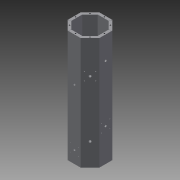
# Autodesk Inventor part: CentralRod_v1.2
Saved by Autodesk Inventor 2015 (Build 190159000, 159)
## iProperties
Created: 2015-09-24
Part Number: CentralRod_v1.2
Material: Generic
Document SubType Name: Modeling
Designer: Stefania
Density: 1 g/cm^3
Appearance: Default
Author: Stefania
Autodesk Inventor part; units mm, degrees
note: some values were not read from the file. Chosen so that the rebuilt part matches the saved one: kept side of "Split6".
ref_plane "XZ Plane" through (0, 0, 0) normal (0, 1, 0) x (-1, 0, 0)
ref_plane "XY Plane" through (0, 0, 0) normal (0, 0, 1) x (1, 0, 0)
sketch "Sketch1" plane through (0, 0, 0) normal (0, 0, 1) x (1, 0, 0)
  line L0 (-15.367, 37.0992) -> (15.367, 37.0992)
  line L1 (15.367, 37.0992) -> (37.0992, 15.367)
  line L2 (37.0992, 15.367) -> (37.0992, -15.367)
  line L3 (37.0992, -15.367) -> (15.367, -37.0992)
  line L4 (15.367, -37.0992) -> (-15.367, -37.0992)
  line L5 (-15.367, -37.0992) -> (-37.0992, -15.367)
  line L6 (-37.0992, -15.367) -> (-37.0992, 15.367)
  line L7 (-37.0992, 15.367) -> (-15.367, 37.0992)
  line L8 (-18.5233, 44.7192) -> (18.5233, 44.7192)
  line L9 (18.5233, 44.7192) -> (44.7192, 18.5233)
  line L10 (44.7192, 18.5233) -> (44.7192, -18.5233)
  line L11 (44.7192, -18.5233) -> (18.5233, -44.7192)
  line L12 (18.5233, -44.7192) -> (-18.5233, -44.7192)
  line L13 (-18.5233, -44.7192) -> (-44.7192, -18.5233)
  line L14 (-44.7192, -18.5233) -> (-44.7192, 18.5233)
  line L15 (-44.7192, 18.5233) -> (-18.5233, 44.7192)
  point P0 (0, 0)
  point P1 (0, 0)
  point P2 (-37.0992, 0)
  point P3 (0, 37.0992)
  dimension "d0" = 30.734
  dimension "d1" = 7.62
  constraints: 32 end point, 2 midpoint, 1 coincident, 1 horizontal alignment, 1 vertical alignment, 24 other
  measures "d0" distance of L0.start L0.end
  measures "d1" distance between parallel lines of L7 L15
extrude "Extrusion1" add sketch "Sketch1" along normal mid plane 304.8
sketch "Sketch2" plane through (18.5233, 44.7192, 152.4) normal (0.7071068, 0.7071068, 0) x (0, 0, -1)
  circle A0 centre (28.956, -18.5233) radius 3.175
  line L0 (0, -37.0466) -> (0, 0) projected
  circle A1 centre (188.976, -18.5233) radius 3.175
  line L1 (304.8, 0) -> (304.8, -37.0466) projected
  point P0 (152.4, -18.5233)
  dimension "d4" = 6.35
  dimension "d5" = 28.956
  dimension "d6" = 6.35
  dimension "d7" = 115.824
  constraints: 2 centre point
  measures "d4" diameter of A0
  measures "d5" distance from line of L0 A0.centre
  measures "d6" diameter of A1
  measures "d7" distance from line of A1.centre L1
extrude "Extrusion2" cut sketch "Sketch2" against normal through all
sketch "Sketch3" plane through (44.7192, -18.5233, 152.4) normal (1, 0, 0) x (0, 0, -1)
  circle A0 centre (57.912, 18.5233) radius 3.175
  line L0 (0, 0) -> (0, 37.0466) projected
  circle A1 centre (217.932, 18.5233) radius 3.175
  point P0 (152.4, 18.5233)
  dimension "d10" = 6.35
  dimension "d11" = 57.912
  dimension "d12" = 6.35
  dimension "d13" = 160.02
  constraints: 2 centre point
  measures "d10" diameter of A0
  measures "d11" distance from line of L0 A0.centre
  measures "d12" diameter of A1
  measures "d13" distance of A1.centre A0.centre
extrude "Extrusion3" cut sketch "Sketch3" against normal through all
sketch "Sketch4" plane through (44.7192, -18.5233, -152.4) normal (0.7071068, -0.7071068, 0) x (0.7071068, 0.7071068, 0)
  circle A0 centre (-18.5233, 217.932) radius 3.175
  line L0 (-37.0466, 304.8) -> (0, 304.8) projected
  circle A1 centre (-18.5233, 57.912) radius 3.175
  point P0 (-18.5233, 152.4)
  dimension "d16" = 6.35
  dimension "d17" = 86.868
  dimension "d18" = 6.35
  dimension "d19" = 160.02
  constraints: 2 centre point
  measures "d16" diameter of A0
  measures "d17" distance from line of L0 A0.centre
  measures "d18" diameter of A1
  measures "d19" distance of A1.centre A0.centre
extrude "Extrusion4" cut sketch "Sketch4" against normal through all
sketch "Sketch5" plane through (-18.5233, -44.7192, 152.4) normal (0, -1, 0) x (1, 0, 0)
  circle A0 centre (18.5233, -115.824) radius 3.175
  circle A1 centre (18.5233, -275.844) radius 3.175
  line L0 (0, 0) -> (37.0466, 0) projected
  point P0 (18.5233, -152.4)
  dimension "d22" = 6.35
  dimension "d23" = 6.35
  dimension "d24" = 115.824
  dimension "d25" = 160.02
  constraints: 2 centre point
  measures "d22" diameter of A0
  measures "d23" diameter of A1
  measures "d24" distance from line of L0 A0.centre
  measures "d25" distance of A1.centre A0.centre
extrude "Extrusion5" cut sketch "Sketch5" against normal through all
sketch "Sketch6" plane through (18.5233, 44.7192, 152.4) normal (0.7071068, 0.7071068, 0) x (0, 0, -1)
  circle A0 centre (17.399, -6.9663) radius 1.016
  circle A1 centre (28.956, -18.5233) radius 3.175 projected
  line L0 (0, 0) -> (304.8, 0) projected
  line L1 (0, -37.0466) -> (0, 0) projected
  circle A2 centre (17.399, -30.0803) radius 1.016
  circle A3 centre (40.513, -6.9663) radius 1.016
  circle A4 centre (40.513, -30.0803) radius 1.016
  point P0 (152.4, -18.5233)
  dimension "d28" = 2.032
  dimension "d29" = 11.557
  dimension "d30" = 11.557
  dimension "d33" = 23.114
  dimension "d40" = 23.114
  constraints: 4 centre point, 1 horizontal, 1 vertical, 6 other
  measures "d28" diameter of A0
  measures "d29" horizontal distance of A1.centre A0.centre
  measures "d30" horizontal distance of A0.centre A1.centre
  measures "d33" distance of A0.centre A2.centre
  measures "d40" distance of A0.centre A3.centre
extrude "Extrusion6" cut sketch "Sketch6" against normal up to surface (7.62 mm away) contours A0 | A2 | A3 | A4
sketch "Sketch7" plane through (-18.5233, -44.7192, -152.4) normal (-0.7071068, -0.7071068, 0) x (0, 0, 1)
  circle A0 centre (127.381, 30.0803) radius 1.016
  circle A1 centre (115.824, 18.5233) radius 3.175 projected
  line L0 (304.8, 37.0466) -> (0, 37.0466) projected
  line L1 (0, 0) -> (0, 37.0466) projected
  circle A2 centre (104.267, 30.0803) radius 1.016
  circle A3 centre (127.381, 6.9663) radius 1.016
  circle A4 centre (104.267, 6.9663) radius 1.016
  point P0 (152.4, 18.5233)
  dimension "d47" = 2.032
  dimension "d48" = 11.557
  dimension "d49" = 11.557
  dimension "d52" = 23.114
  dimension "d59" = 23.114
  constraints: 4 centre point, 1 horizontal, 1 vertical, 6 other
  measures "d47" diameter of A0
  measures "d48" horizontal distance of A0.centre A1.centre
  measures "d49" horizontal distance of A1.centre A0.centre
  measures "d52" distance of A0.centre A2.centre
  measures "d59" distance of A2.centre A4.centre
extrude "Extrusion7" cut sketch "Sketch7" against normal blind 7.62 contours A0 | A2 | A3 | A4
sketch "Sketch8" plane through (-44.7192, 18.5233, 152.4) normal (-0.7071068, 0.7071068, 0) x (0.7071068, 0.7071068, 0)
  circle A0 centre (6.9663, 258.445) radius 1.016
  circle A1 centre (18.5233, 246.888) radius 3.175 projected
  line L0 (0, 0) -> (0, 304.8) projected
  line L1 (0, 304.8) -> (37.0466, 304.8) projected
  circle A2 centre (30.0803, 258.445) radius 1.016
  circle A3 centre (6.9663, 235.331) radius 1.016
  circle A4 centre (30.0803, 235.331) radius 1.016
  point P0 (18.5233, 152.4)
  dimension "d66" = 11.557
  dimension "d67" = 11.557
  dimension "d70" = 23.114
  dimension "d77" = 23.114
  dimension "d82" = 2.032
  constraints: 4 centre point, 1 horizontal, 1 vertical, 6 other
  measures "d66" horizontal distance of A1.centre A0.centre
  measures "d67" horizontal distance of A1.centre A0.centre
  measures "d70" distance of A0.centre A2.centre
  measures "d77" distance of A0.centre A3.centre
  measures "d82" diameter of A0
extrude "Extrusion8" cut sketch "Sketch8" against normal blind 7.62 contours A0 | A2 | A3 | A4
sketch "Sketch9" plane through (44.7192, -18.5233, -152.4) normal (0.7071068, -0.7071068, 0) x (0.7071068, 0.7071068, 0)
  line L0 (0, 304.8) -> (0, 0) projected
  line L1 (-37.0466, 304.8) -> (0, 304.8) projected
  circle A0 centre (-6.9663, 229.489) radius 1.016
  circle A1 centre (-18.5233, 217.932) radius 3.175 projected
  circle A2 centre (-6.9663, 206.375) radius 1.016
  circle A3 centre (-30.0803, 229.489) radius 1.016
  circle A4 centre (-30.0803, 206.375) radius 1.016
  point P0 (-18.5233, 152.4)
  dimension "d85" = 2.032
  dimension "d86" = 11.557
  dimension "d87" = 11.557
  dimension "d90" = 23.114
  dimension "d97" = 23.114
  constraints: 4 centre point, 1 horizontal, 1 vertical, 6 other
  measures "d85" diameter of A0
  measures "d86" horizontal distance of A0.centre A1.centre
  measures "d87" horizontal distance of A1.centre A0.centre
  measures "d90" distance of A0.centre A2.centre
  measures "d97" distance of A0.centre A3.centre
extrude "Extrusion9" cut sketch "Sketch9" against normal blind 7.62 contours A0 | A2 | A3 | A4
sketch "Sketch10" plane through (-44.7192, -18.5233, 152.4) normal (-1, 0, 0) x (0, 0, 1)
  line L0 (0, 0) -> (-304.8, 0) projected
  line L1 (0, 37.0466) -> (0, 0) projected
  circle A0 centre (-57.912, 18.5233) radius 3.175 projected
  circle A1 centre (-69.469, 6.9663) radius 1.016
  circle A2 centre (-46.355, 6.9663) radius 1.016
  circle A3 centre (-69.469, 30.0803) radius 1.016
  circle A4 centre (-46.355, 30.0803) radius 1.016
  point P0 (-152.4, 18.5233)
  dimension "d104" = 2.032
  dimension "d105" = 11.557
  dimension "d106" = 11.557
  dimension "d109" = 23.114
  dimension "d116" = 23.114
  constraints: 4 centre point, 1 horizontal, 1 vertical, 6 other
  measures "d104" diameter of A1
  measures "d105" horizontal distance of A0.centre A1.centre
  measures "d106" horizontal distance of A0.centre A1.centre
  measures "d109" distance of A1.centre A2.centre
  measures "d116" distance of A2.centre A4.centre
extrude "Extrusion10" cut sketch "Sketch10" against normal blind 7.62 contours A1 | A2 | A3 | A4
sketch "Sketch11" plane through (44.7192, -18.5233, 152.4) normal (1, 0, 0) x (0, 0, -1)
  line L0 (304.8, 37.0466) -> (304.8, 0) projected
  line L1 (0, 0) -> (304.8, 0) projected
  circle A0 centre (217.932, 18.5233) radius 3.175 projected
  circle A1 centre (229.489, 6.9663) radius 1.016
  circle A2 centre (206.375, 6.9663) radius 1.016
  circle A3 centre (229.489, 30.0803) radius 1.016
  circle A4 centre (206.375, 30.0803) radius 1.016
  point P0 (152.4, 18.5233)
  dimension "d123" = 2.032
  dimension "d124" = 11.557
  dimension "d125" = 11.557
  dimension "d128" = 23.114
  dimension "d135" = 23.114
  constraints: 4 centre point, 1 horizontal, 1 vertical, 6 other
  measures "d123" diameter of A1
  measures "d124" horizontal distance of A0.centre A1.centre
  measures "d125" horizontal distance of A0.centre A1.centre
  measures "d128" distance of A1.centre A2.centre
  measures "d135" distance of A1.centre A3.centre
extrude "Extrusion11" cut sketch "Sketch11" against normal blind 7.62 contours A1 | A2 | A3 | A4
sketch "Sketch12" plane through (-18.5233, -44.7192, 152.4) normal (0, -1, 0) x (1, 0, 0)
  line L0 (0, 0) -> (0, -304.8) projected
  line L1 (37.0466, -304.8) -> (0, -304.8) projected
  circle A0 centre (18.5233, -275.844) radius 3.175 projected
  circle A1 centre (6.9663, -287.401) radius 1.016
  circle A2 centre (6.9663, -264.287) radius 1.016
  circle A3 centre (30.0803, -287.401) radius 1.016
  circle A4 centre (30.0803, -264.287) radius 1.016
  point P0 (18.5233, -152.4)
  dimension "d142" = 2.032
  dimension "d143" = 11.557
  dimension "d144" = 11.557
  dimension "d147" = 23.114
  dimension "d154" = 23.114
  constraints: 4 centre point, 1 horizontal, 1 vertical, 6 other
  measures "d142" diameter of A1
  measures "d143" horizontal distance of A0.centre A1.centre
  measures "d144" horizontal distance of A0.centre A1.centre
  measures "d147" distance of A1.centre A2.centre
  measures "d154" distance of A1.centre A3.centre
extrude "Extrusion12" cut sketch "Sketch12" against normal blind 7.62 contours A1 | A2 | A3 | A4
sketch "Sketch13" plane through (-18.5233, 44.7192, 152.4) normal (0, 1, 0) x (1, 0, 0)
  line L0 (0, 304.8) -> (0, 0) projected
  line L1 (37.0466, 0) -> (0, 0) projected
  circle A0 centre (18.5233, 115.824) radius 3.175 projected
  circle A1 centre (6.9663, 104.267) radius 1.016
  circle A2 centre (6.9663, 127.381) radius 1.016
  circle A3 centre (30.0803, 104.267) radius 1.016
  circle A4 centre (30.0803, 127.381) radius 1.016
  point P0 (18.5233, 152.4)
  dimension "d161" = 2.032
  dimension "d162" = 11.557
  dimension "d163" = 11.557
  dimension "d166" = 23.114
  dimension "d173" = 23.114
  constraints: 4 centre point, 1 horizontal, 1 vertical, 6 other
  measures "d161" diameter of A1
  measures "d162" horizontal distance of A0.centre A1.centre
  measures "d163" horizontal distance of A0.centre A1.centre
  measures "d166" distance of A1.centre A2.centre
  measures "d173" distance of A1.centre A3.centre
extrude "Extrusion13" cut sketch "Sketch13" against normal blind 7.62 contours A1 | A2 | A3 | A4
sketch "Sketch14" plane through (0, 0, -152.4) normal (0, 0, -1) x (-1, 0, 0)
  circle A0 centre (0, 40.9092) radius 1.7526
  circle A1 centre (-28.9272, 28.9272) radius 1.7526
  circle A2 centre (28.9272, 28.9272) radius 1.7526
  circle A3 centre (-40.9092, 0) radius 1.7526
  circle A4 centre (40.9092, 0) radius 1.7526
  circle A5 centre (0, -40.9092) radius 1.7526
  circle A6 centre (-28.9272, -28.9272) radius 1.7526
  circle A7 centre (28.9272, -28.9272) radius 1.7526
  point P0 (0, 0)
  dimension "d180" = 3.5052
  dimension "d184" = 45
  dimension "d188" = 45
  dimension "d192" = 45
  dimension "d196" = 45
  constraints: 8 centre point, 12 other
  measures "d180" diameter of A0
extrude "Extrusion14" cut sketch "Sketch14" against normal blind 12.7
thread "Thread1" size "6-32 UNC" class "2B" standard "ANSI Unified Screw Threads" full length
thread "Thread2" size "6-32 UNC" class "2B" standard "ANSI Unified Screw Threads" full length
thread "Thread3" size "6-32 UNC" class "2B" standard "ANSI Unified Screw Threads" full length
thread "Thread4" size "6-32 UNC" class "2B" standard "ANSI Unified Screw Threads" full length
thread "Thread5" size "6-32 UNC" class "2B" standard "ANSI Unified Screw Threads" full length
thread "Thread6" size "6-32 UNC" class "2B" standard "ANSI Unified Screw Threads" full length
thread "Thread7" size "6-32 UNC" class "2B" standard "ANSI Unified Screw Threads" full length
thread "Thread8" size "6-32 UNC" class "2B" standard "ANSI Unified Screw Threads" full length
mirror "Mirror1" about plane through (0, 0, 0) normal (0, 0, 1) of "Extrusion14"
thread "Thread9" size "6-32 UNC" class "2B" standard "ANSI Unified Screw Threads" full length
thread "Thread10" size "6-32 UNC" class "2B" standard "ANSI Unified Screw Threads" full length
thread "Thread11" size "6-32 UNC" class "2B" standard "ANSI Unified Screw Threads" full length
thread "Thread12" size "6-32 UNC" class "2B" standard "ANSI Unified Screw Threads" full length
thread "Thread13" size "6-32 UNC" class "2B" standard "ANSI Unified Screw Threads" full length
thread "Thread14" size "6-32 UNC" class "2B" standard "ANSI Unified Screw Threads" full length
thread "Thread15" size "6-32 UNC" class "2B" standard "ANSI Unified Screw Threads" full length
thread "Thread16" size "6-32 UNC" class "2B" standard "ANSI Unified Screw Threads" full length
sketch "Sketch15" plane through (0, 0, -152.4) normal (0, 0, -1) x (-1, 0, 0)
  circle A0 centre (28.9272, -28.9272) radius 1.7526 projected
  circle A1 centre (40.9092, 0) radius 1.7526 projected
  circle A2 centre (28.9272, 28.9272) radius 1.7526 projected
  circle A3 centre (0, 40.9092) radius 1.7526 projected
  circle A4 centre (-28.9272, 28.9272) radius 1.7526 projected
  circle A5 centre (-40.9092, 0) radius 1.7526 projected
  circle A6 centre (0, -40.9092) radius 1.7526 projected
  circle A7 centre (-28.9272, -28.9272) radius 1.7526 projected
  line L0 (-37.0992, 15.367) -> (-15.367, 37.0992) projected
  line L1 (-15.367, 37.0992) -> (15.367, 37.0992) projected
  line L2 (15.367, 37.0992) -> (37.0992, 15.367) projected
  line L3 (37.0992, 15.367) -> (37.0992, -15.367) projected
  line L4 (37.0992, -15.367) -> (15.367, -37.0992) projected
  line L5 (15.367, -37.0992) -> (-15.367, -37.0992) projected
  line L6 (-15.367, -37.0992) -> (-37.0992, -15.367) projected
  line L7 (-37.0992, -15.367) -> (-37.0992, 15.367) projected
  line L8 (18.5233, 44.7192) -> (-18.5233, 44.7192) projected
  line L9 (-18.5233, 44.7192) -> (-44.7192, 18.5233) projected
  line L10 (-44.7192, 18.5233) -> (-44.7192, -18.5233) projected
  line L11 (-44.7192, -18.5233) -> (-18.5233, -44.7192) projected
  line L12 (-18.5233, -44.7192) -> (18.5233, -44.7192) projected
  line L13 (18.5233, -44.7192) -> (44.7192, -18.5233) projected
  line L14 (44.7192, -18.5233) -> (44.7192, 18.5233) projected
  line L15 (44.7192, 18.5233) -> (18.5233, 44.7192) projected
  point P0 (0, 0)
extrude "Extrusion15" add sketch "Sketch15" along normal blind 6.35
sketch "Sketch16" plane through (0, 0, 152.4) normal (0, 0, 1) x (1, 0, 0)
  circle A0 centre (-28.9272, -28.9272) radius 1.7526 projected
  circle A1 centre (-40.9092, 0) radius 1.7526 projected
  circle A2 centre (-28.9272, 28.9272) radius 1.7526 projected
  circle A3 centre (0, 40.9092) radius 1.7526 projected
  circle A4 centre (28.9272, 28.9272) radius 1.7526 projected
  circle A5 centre (40.9092, 0) radius 1.7526 projected
  circle A6 centre (0, -40.9092) radius 1.7526 projected
  circle A7 centre (28.9272, -28.9272) radius 1.7526 projected
  line L0 (15.367, 37.0992) -> (37.0992, 15.367) projected
  line L1 (37.0992, 15.367) -> (37.0992, -15.367) projected
  line L2 (37.0992, -15.367) -> (15.367, -37.0992) projected
  line L3 (15.367, -37.0992) -> (-15.367, -37.0992) projected
  line L4 (-15.367, -37.0992) -> (-37.0992, -15.367) projected
  line L5 (-37.0992, -15.367) -> (-37.0992, 15.367) projected
  line L6 (-37.0992, 15.367) -> (-15.367, 37.0992) projected
  line L7 (-15.367, 37.0992) -> (15.367, 37.0992) projected
  line L8 (18.5233, 44.7192) -> (-18.5233, 44.7192) projected
  line L9 (-18.5233, 44.7192) -> (-44.7192, 18.5233) projected
  line L10 (-44.7192, 18.5233) -> (-44.7192, -18.5233) projected
  line L11 (-44.7192, -18.5233) -> (-18.5233, -44.7192) projected
  line L12 (-18.5233, -44.7192) -> (18.5233, -44.7192) projected
  line L13 (18.5233, -44.7192) -> (44.7192, -18.5233) projected
  line L14 (44.7192, -18.5233) -> (44.7192, 18.5233) projected
  line L15 (44.7192, 18.5233) -> (18.5233, 44.7192) projected
  point P0 (0, 0)
extrude "Extrusion16" add sketch "Sketch16" along normal blind 6.35
ref_plane "Work Plane1" through (15.367, 37.0992, -152.4) normal (0.9238795, -0.3826834, 0) x (0, 0, -1)
split body "Split1" result two bodies by plane through (15.367, 37.0992, -152.4) normal (0.9238795, -0.3826834, 0) first body at (-0.1276, -44.2192, 119.076)
ref_plane "Work Plane2" through (-15.367, 37.0992, 152.4) normal (0.9238795, 0.3826834, 0) x (0, 0, 1)
split body "Split2" result two bodies by plane through (-15.367, 37.0992, 152.4) normal (0.9238795, 0.3826834, 0) bodies 3 first body at (3.8115, 44.2192, 122.2139)
ref_plane "Work Plane3" through (-37.0992, 15.367, 152.4) normal (0.3826834, 0.9238795, 0) x (0, 0, 1)
split body "Split3" result two bodies by plane through (-37.0992, 15.367, 152.4) normal (0.3826834, 0.9238795, 0) bodies 5 first body at (-31.1775, 31.3579, 128.728)
ref_plane "Work Plane4" through (-37.0992, -15.367, 152.4) normal (-0.3826834, 0.9238795, 0) x (0, 0, 1)
split body "Split4" result two bodies by plane through (-37.0992, -15.367, 152.4) normal (-0.3826834, 0.9238795, 0) bodies 7 first body at (-44.2192, 0, -128.7357)
split body "Split5" result two bodies by plane through (-37.0992, -15.367, 152.4) normal (-0.3826834, 0.9238795, 0) bodies 2 first body at (31.2677, 31.2677, -119.0837)
split body "Split6" result two bodies by plane through (-37.0992, 15.367, 152.4) normal (0.3826834, 0.9238795, 0) bodies 11 first body at (-0.1276, -44.2192, 119.076)
split body "Split7" result two bodies by plane through (-15.367, 37.0992, 152.4) normal (0.9238795, 0.3826834, 0) bodies 12 first body at (31.3579, -31.1775, 4.8656)
equation "\"d8\" = d4"
body "Solid4"
body "Solid6"
body "Solid8"
body "Solid9"
body "Solid10"
body "Solid13"
body "Solid14"
body "Solid15"
